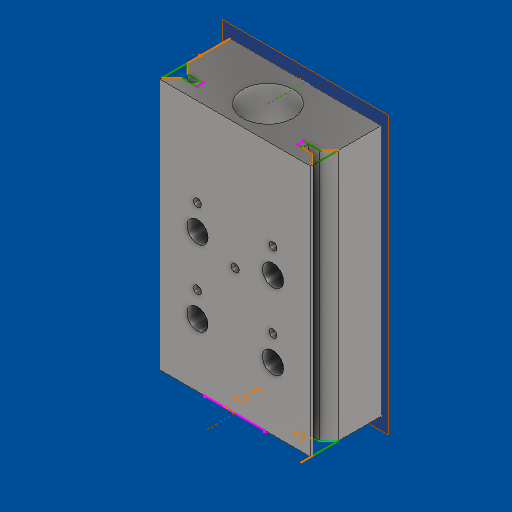
# Autodesk Inventor part: Platform
Saved by Autodesk Inventor 2025.1 (Build 291241000, 241)
## iProperties
Created: 2024-12-17
Part Number: Platform
Material: Steel, Carbon
Document SubType Name: Modeling
Designer: konch
Density: 7.85 g/cm^3
Appearance: Semi-Polished
Mass: 150.059 g
Surface Area: 69.2478 cm^2
Volume: 19.1159 cm^3
Description: C55
Author: konch
Autodesk Inventor part; units mm, degrees
ref_plane "YZ Plane" through (0, 0, 0) normal (1, 0, 0) x (0, 1, 0)
ref_plane "XZ Plane" through (0, 0, 0) normal (0, 1, 0) x (-1, 0, 0)
ref_plane "XY Plane" through (0, 0, 0) normal (0, 0, 1) x (1, 0, 0)
sketch "Sketch1" plane through (0, 0, 0) normal (0, 0, 1) x (1, 0, 0)
  line L0 (0, 0) -> (30, 0)
  line L1 (30, 0) -> (30, 50)
  line L2 (30, 50) -> (0, 50)
  line L3 (0, 50) -> (0, 0)
  dimension "d0" = 30
  dimension "d1" = 50
  constraints: 8 end point, 3 perpendicular, 1 horizontal
  measures "d0" distance of L0.start L0.end
  measures "d1" distance of L0.end L1.end
extrude "Extrusion1" add sketch "Sketch1" along normal blind 10
sketch "Sketch2" plane through (0, 0, 0) normal (0, -1, 0) x (1, 0, 0)
  line L0 (30, 0) -> (30, 10) projected
  line L1 (30, 0) -> (30, 1.5)
  line L2 (15, 0) -> (15, 12.0836) construction
  line L3 (30, 10) -> (30, 9) construction
  line L4 (30, 9) -> (-1.4785, 9) construction
  line L5 (27.4716, 5) -> (-0.9945, 5) construction
  line L6 (30, 5) -> (30.3, 5) construction
  line L7 (28.0716, 4.4) -> (30, 2.4716)
  line L8 (28.0716, 5.6) -> (30, 7.5284)
  line L9 (30, 5) -> (30, 5.6) construction
  line L10 (28.0716, 5.6) -> (25, 5.6)
  line L11 (25, 5.6) -> (25, 4.4)
  line L12 (25, 4.4) -> (28.0716, 4.4)
  arc A0 (30, 6.9774) -> (28.8858, 6.4142) centre (30.3, 5) ccw construction
  arc A1 (28.3921, 4.4) -> (28.8858, 3.5858) centre (30.3, 5) ccw construction
  line L13 (1.9284, 4.4) -> (0, 2.4716)
  line L14 (1.9284, 5.6) -> (0, 7.5284)
  line L15 (1.9284, 5.6) -> (5, 5.6)
  line L16 (5, 5.6) -> (5, 4.4)
  line L17 (5, 4.4) -> (1.9284, 4.4)
  line L18 (30, 10) -> (0, 10) projected
  line L19 (0, 0) -> (0, 10) projected
  line L20 (0, 10) -> (0, 0)
  line L21 (30, 0) -> (30, -3)
  line L22 (30, -3) -> (0, -3)
  line L23 (0, -3) -> (0, 0)
  line L24 (30, 0) -> (0, 0) projected
  line L25 (0, 0) -> (30, 0)
  circle A2 centre (15, 5) radius 1.5
  line L26 (4, 4.4) -> (4, 5.6)
  line L27 (25, 4.4) -> (26, 4.4)
  line L28 (26, 4.4) -> (26, 5.6)
  line L29 (25, 5.6) -> (25, 4.4)
  point P0 (4, 5)
  dimension "d4" = 1.5
  dimension "d7" = 1
  dimension "d9" = 0.3
  dimension "d11" = 90
  dimension "d12" = 0.6
  dimension "d13" = 5
  dimension "d14" = 1.2
  dimension "d27" = 3
  dimension "d31" = 3
  dimension "d90" = 5
  dimension "d91" = 4
  dimension "d94" = 1
  constraints: 52 end point, 17 point on line, 9 perpendicular, 6 symmetric about line, 4 point on circle, 3 centre point, 3 collinear, 2 tangent, 1 coincident, 1 horizontal, 1 midpoint, 1 vertical
  measures "d4" distance of L0.start L1.end
  measures "d7" distance of L0.end L3.end
  measures "d9" distance of L6.start L6.end
  measures "d11" angle of L7 L8
  measures "d12" distance of L6.start L9.end
  measures "d13" distance of L9.end L10.end
  measures "d14" distance of L10.end L11.end
  measures "d27" distance of L0.start L21.end
  measures "d31" diameter of A2
  measures "d90" distance between parallel lines of L19 L16
  measures "d91" distance from line of L19 point (4, 5)
  measures "d94" distance of L11.end L27.end
extrude "Extrusion3" cut sketch "Sketch2" against normal blind 50 contours L7 L12 L28 L10 L8 L0 | L19 L14 L15 L26 L17 L13
sketch "Sketch4" plane through (0, 0, 0) normal (0, -1, 0) x (1, 0, 0)
  line L0 (30, 0) -> (0, 0) projected
  line L1 (30, 0) -> (0, 0)
  line L2 (0, 0) -> (0, -6)
  line L3 (0, -6) -> (30, -6)
  line L4 (30, -6) -> (30, 0)
  dimension "d28" = 6
  constraints: 8 end point, 3 perpendicular, 1 collinear
  measures "d28" distance of L0.end L2.end
extrude "Extrusion5" add sketch "Sketch4" against normal blind 50
sketch "Sketch5" plane through (1.9284, 0, 5.6) normal (0, -1, 0) x (1, 0, 0)
  line L0 (23.0716, -1.2) -> (23.0716, 0) projected
  line L1 (23.0716, -0.6) -> (3.0716, -0.6) construction
  line L2 (19.0716, 2.4) -> (7.0716, 2.4) projected
  line L3 (13.0716, 2.4) -> (13.0716, -11.6) construction
  line L4 (-1.9284, -11.6) -> (28.0716, -11.6) projected
  line L5 (13.0716, 2.4) -> (13.0716, -4.1)
  line L6 (13.0716, -4.1) -> (-1.9284, -4.1) construction
  line L7 (-1.9284, -11.6) -> (-1.9284, -3.1284) construction
  point P0 (-1.9284, -5.6)
  dimension "d33" = 6.5
  constraints: 8 end point, 3 midpoint, 2 horizontal, 2 point on line, 1 coincident
  measures "d33" distance of L3.start L5.end
ref_plane "Work Plane1" through (30, 0, -6) normal (0, 0, -1) x (-1, 0, 0)
sketch "Sketch7" plane through (25, 50, 5.6) normal (0, 1, 0) x (1, 0, 0)
  line L0 (-25, -1.9284) -> (-23.0716, 0) projected
  line L1 (-25, 11.6) -> (-25, 3.1284) projected
  line L2 (-25, -1.9284) -> (-25, 3.1284)
  line L3 (-23.0716, 1.2) -> (-25, 3.1284) projected
  line L4 (-25, 3.1284) -> (-23.0716, 1.2)
  line L5 (-20, 0) -> (-20, 1.2) projected
  line L6 (-23.0716, 1.2) -> (-20, 1.2)
  line L7 (-20, 1.2) -> (-20, 0)
  line L8 (-20, 0) -> (-23.0716, 0)
  line L9 (-23.0716, 0) -> (-25, -1.9284)
  line L10 (0, 0) -> (0, 1.2) projected
  line L11 (0, 0) -> (0, 1.2)
  line L12 (0, 1.2) -> (3.4081, 1.2)
  line L13 (3.0716, 1.2) -> (5, 3.1284) projected
  line L14 (5, 3.1284) -> (3.0716, 1.2)
  line L15 (3.0716, 0) -> (1, 0) projected
  line L16 (0, 0) -> (3.0716, 0)
  line L17 (5, -1.9284) -> (3.0716, 0) projected
  line L18 (3.0716, 0) -> (5, -1.9284)
  line L19 (5, -1.9284) -> (5, 3.1284)
  point P0 (-25, 5.6)
  constraints: 24 end point, 6 collinear, 5 perpendicular, 1 vertical
sketch "Sketch8" plane through (1.9284, 0, 5.6) normal (0, -1, 0) x (1, 0, 0)
  line L0 (28.0716, 1.9284) -> (28.0716, 4.4) projected
  line L1 (28.0716, 1.9284) -> (28.0716, -3.1284)
  line L2 (28.0716, -3.1284) -> (26.1431, -1.2)
  line L3 (23.0716, -1.2) -> (23.0716, 0) projected
  line L4 (26.1431, -1.2) -> (23.0716, -1.2)
  line L5 (23.0716, -1.2) -> (23.0716, 0)
  line L6 (23.0716, 0) -> (26.1431, 0)
  line L7 (26.1431, 0) -> (28.0716, 1.9284)
  line L8 (13.0716, -3.7758) -> (13.0716, 8.1492) construction
  line L9 (-1.9284, -3.1284) -> (0, -1.2)
  line L10 (-1.9284, 1.9284) -> (-1.9284, -3.1284)
  line L11 (3.0716, -1.2) -> (3.0716, 0)
  line L12 (0, -1.2) -> (3.0716, -1.2)
  line L13 (3.0716, 0) -> (0, 0)
  line L14 (0, 0) -> (-1.9284, 1.9284)
  line L15 (23.0716, -1.2) -> (24.0716, -1.2)
  line L16 (24.0716, -1.2) -> (24.0716, 0)
  line L17 (23.0716, 0) -> (23.0716, -1.2)
  point P0 (-1.9284, -5.6)
  dimension "d93" = 1
  constraints: 32 end point, 6 symmetric about line, 4 perpendicular, 2 equal length, 2 point on line, 2 vertical
  measures "d93" distance of L3.start L15.end
sketch "Sketch10" plane through (30, 0, -6) normal (0, 0, -1) x (-1, 0, 0)
  line L0 (0, 50) -> (30, 50) construction
  line L1 (0, 50) -> (7.5, 50) construction
  line L2 (7.5, 50) -> (7.5, 32.5) construction
  line L3 (30, 50) -> (22.5, 50) construction
  line L4 (22.5, 50) -> (22.5, 32.5) construction
  line L5 (30, 0) -> (0, 0) construction
  line L6 (0, 0) -> (7.5, 0) construction
  line L7 (7.5, 0) -> (7.5, 17.5) construction
  line L8 (30, 0) -> (22.5, 0) construction
  line L9 (22.5, 0) -> (22.5, 17.5) construction
  line L10 (21, 50) -> (9, 50) construction
  line L11 (15, 50) -> (15, 25) construction
  line L12 (0, 0) -> (0, 50) construction
  line L13 (15, 25) -> (0, 25)
  point P0 (0, 5)
  point P1 (0, 45)
  dimension "d53" = 7.5
  dimension "d54" = 17.5
  dimension "d55" = 7.5
  dimension "d56" = 17.5
  dimension "d57" = 7.5
  dimension "d58" = 17.5
  dimension "d59" = 7.5
  dimension "d60" = 17.5
  constraints: 20 end point, 7 coincident, 4 perpendicular, 4 point on line, 2 midpoint, 1 parallel
  measures "d53" distance of L0.start L1.end
  measures "d54" distance of L1.end L2.end
  measures "d55" distance of L0.end L3.end
  measures "d56" distance of L3.end L4.end
  measures "d57" distance of L5.end L6.end
  measures "d58" distance of L6.end L7.end
  measures "d59" distance of L5.start L8.end
  measures "d60" distance of L8.end L9.end
hole "Hole2" at (22.5, 17.5, -6) at (7.5, 17.5, -6) at (7.5, 32.5, -6) at (22.5, 32.5, -6) at (15, 25, -6) direction (0, 0, 1) diameter 1.567 end through all thread size "M2x0.4" class "6H" standard "ISO Metric profile"
sketch "Sketch11" plane through (30, 0, -6) normal (0, 0, -1) x (-1, 0, 0)
  circle A0 centre (22.5, 32.5) radius 0.7835 projected
  circle A1 centre (7.5, 32.5) radius 0.7835 projected
  point P0 (30, 0)
  point P1 (22.5, 12.5)
  point P2 (7.5, 12.5)
  point P3 (22.5, 27.5)
  point P4 (7.5, 27.5)
  dimension "d68" = 20
  dimension "d76" = 15
  constraints: 4 vertical alignment, 2 horizontal alignment
  measures "d68" distance of A1.centre point (7.5, 12.5)
  measures "d76" distance of point (22.5, 27.5) point (22.5, 12.5)
hole "Hole3" at (7.5, 12.5, -6) at (22.5, 12.5, -6) at (7.5, 27.5, -6) at (22.5, 27.5, -6) direction (0, 0, 1) diameter 4.2 end through all
chamfer "Chamfer1" distance 0.3 angle 45 5 edges at (7.5, 31.7165, -6) (7.5, 16.7165, -6) (22.5, 16.7165, -6) (22.5, 31.7165, -6) (15, 24.2165, -6)
sketch "Sketch12" plane through (0, 0, 10) normal (0, -1, 0) x (1, 0, 0)
  line L0 (30, -2.4716) -> (30, 0) projected
  line L1 (30, 0) -> (30, -2)
  line L2 (30, -2) -> (0, -2)
  line L3 (30, -2) -> (30, 0)
  line L4 (0, 0) -> (30, 0) projected
  line L5 (0, 0) -> (0, -2)
  line L6 (0, -2.4716) -> (0, 0) projected
  point P0 (0, -10)
  dimension "d80" = 2
  constraints: 8 end point, 2 collinear, 1 perpendicular, 1 point on line
  measures "d80" distance of L0.end L1.end
extrude "Extrusion10" cut sketch "Sketch12" against normal through all
chamfer "Chamfer2" distance 0.3 angle 45 1 edges at (15, 24.2165, -5.7)
sketch "Sketch13" plane through (25, 50, 5.6) normal (0, 1, 0) x (1, 0, 0)
  line L0 (-8.9165, 11.6) -> (-11.0835, 11.6) construction
  line L1 (-10, 11.6) -> (-10, 3.4303) construction
  point P0 (-25, 5.6)
  constraints: 2 end point, 1 midpoint, 1 vertical
sketch "Sketch14" plane through (25, 50, 5.6) normal (0, 1, 0) x (1, 0, 0)
  line L0 (-10.7835, -2.4) -> (-9.2165, -2.4) projected
  line L1 (-10, -2.4) -> (-10, 4.1)
  circle A0 centre (-10, 4.1) radius 5
  point P0 (-25, 5.6)
  dimension "d86" = 6.5
  dimension "d87" = 10
  constraints: 2 end point, 1 centre point, 1 coincident, 1 midpoint, 1 vertical
  measures "d86" distance of L1.start L1.end
  measures "d87" diameter of A0
extrude "Extrusion11" cut sketch "Sketch14" against normal blind 17
sketch "Sketch15" plane through (25, 0, 4.4) normal (0, -1, 0) x (1, 0, 0)
  line L0 (3.0716, 0) -> (1, 0) projected
  line L1 (0, 0) -> (1, 0)
  line L2 (1, 0) -> (1, 1.2)
  line L3 (1, 1.2) -> (3.0716, 1.2) projected
  line L4 (1, 0) -> (0, 0)
  line L5 (0, 0) -> (0, 1.2) projected
  line L6 (0, 1.2) -> (1, 1.2)
  point P0 (-25, -4.4)
  dimension "d92" = 1
  constraints: 10 end point, 2 collinear, 1 perpendicular
  measures "d92" distance of L1.start L0.end
equation "\"d54\" = d56"
equation "\"d58\" = d56"
equation "\"d60\" = d56"
body "Solid1"
